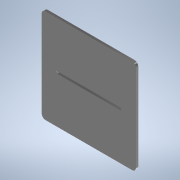
# Autodesk Inventor part: Slit
Saved by Autodesk Inventor 2020 (Build 240168000, 168)
## iProperties
Created: 2019-09-09
Part Number: Slit
Material: Stainless Steel, Austenitic
Document SubType Name: Sheet Metal
Designer: vmiguel
Density: 8 g/cm^3
Sheet Metal Rule: Default_mm
Appearance: Semi-Polished
Author: vmiguel
Autodesk Inventor part; units mm, degrees
ref_plane "YZ Plane" through (0, 0, 0) normal (1, 0, 0) x (0, 1, 0)
ref_plane "XZ Plane" through (0, 0, 0) normal (0, 1, 0) x (-1, 0, 0)
ref_plane "XY Plane" through (0, 0, 0) normal (0, 0, 1) x (1, 0, 0)
sketch "Sketch1" plane through (0, 0, 0) normal (0, 0, 1) x (1, 0, 0)
  line L0 (-5.5, 6) -> (5.5, 6)
  line L1 (6, 5.5) -> (6, -5.5)
  line L2 (5.5, -6) -> (-5.5, -6)
  line L3 (-6, -5.5) -> (-6, 5.5)
  line L4 (-6, 6) -> (6, -6) construction
  line L5 (6, 6) -> (-6, -6) construction
  line L6 (-4, 0) -> (4, 0) construction
  line L7 (-4, -0.15) -> (4, -0.15)
  line L8 (4, 0.15) -> (-4, 0.15)
  arc A0 (-4, 0.15) -> (-4, -0.15) centre (-4, 0) ccw
  arc A1 (4, -0.15) -> (4, 0.15) centre (4, 0) ccw
  arc A2 (-5.5, 6) -> (-6, 5.5) centre (-5.5, 5.5) ccw
  arc A3 (-6, -5.5) -> (-5.5, -6) centre (-5.5, -5.5) ccw
  arc A4 (5.5, -6) -> (6, -5.5) centre (5.5, -5.5) ccw
  arc A5 (6, 5.5) -> (5.5, 6) centre (5.5, 5.5) ccw
  point P0 (0, 0)
  dimension "d0" = 12
  dimension "d1" = 12
  dimension "d2" = 4
  dimension "d3" = 0.3
  dimension "d4" = 0.5
  measures "d0" distance of L4.end L5.end
  measures "d1" distance of L5.start L4.end
  measures "d2" distance of point (0, 0) L6.end
  measures "d3" diameter of A1
  measures "d4" radius of A2
extrude "Plate1" add sketch "Sketch1" along normal blind 0.3
equation "\"d5\" = Thickness"
equation "\"BendRadius\" = Thickness"
equation "\"BendReliefWidth\" = Thickness"
equation "\"BendReliefDepth\" = 0.5 * Thickness"
equation "\"CornerReliefSize\" = 4 * Thickness"
equation "\"MinimumRemnant\" = 2 * Thickness"
equation "\"TransitionRadius\" = BendRadius"
equation "\"JacobiRadiusSize\" = BendRadius"
equation "\"GapSize\" = Thickness"
equation "\"Thickness\" = 0.3"
body "Solid1"
